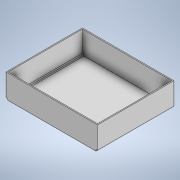
# Autodesk Inventor part: soap-collector
Saved by Autodesk Inventor 2020.2 (Build 242310000, 310)
## iProperties
Created: 2020-03-31
Part Number: soap-collector
Material: Generic
Document SubType Name: Modeling
Designer: iamin
Density: 1 g/cm^3
Appearance: Default
Author: iamin
Autodesk Inventor part; units mm, degrees
ref_plane "YZ Plane" through (0, 0, 0) normal (1, 0, 0) x (0, 1, 0)
ref_plane "XZ Plane" through (0, 0, 0) normal (0, 1, 0) x (-1, 0, 0)
ref_plane "XY Plane" through (0, 0, 0) normal (0, 0, 1) x (1, 0, 0)
sketch "Sketch1" plane through (0, 0, 0) normal (0, 0, 1) x (1, 0, 0)
  line L0 (-43.15, -11.5) -> (44.65, -11.5)
  line L1 (44.65, -11.5) -> (44.65, 11.5)
  line L2 (44.65, 11.5) -> (-44.65, 11.5)
  line L3 (-44.65, 11.5) -> (-44.65, -11.5)
  line L4 (-44.65, -11.5) -> (44.65, 11.5) construction
  line L5 (44.65, -11.5) -> (-44.65, 11.5) construction
  line L6 (-44.65, -11.5) -> (-44.65, -10)
  line L7 (-44.65, -10) -> (-43.15, -10)
  line L8 (-43.15, -10) -> (-43.15, -11.5)
  line L9 (0, 0) -> (0, -4.954)
  line L10 (44.65, -11.5) -> (-44.65, -11.5)
  line L11 (44.65, 11.5) -> (44.65, -11.5)
  line L12 (44.65, -11.5) -> (-44.65, 11.5) construction
  line L13 (44.65, -11.5) -> (44.65, -10)
  line L14 (44.65, -10) -> (43.15, -10)
  line L15 (43.15, -10) -> (43.15, -11.5)
  dimension "d0" = 89.3
  dimension "d1" = 23
  dimension "d3" = 1.5
  constraints: 32 end point, 7 symmetric about line, 3 perpendicular, 3 point on line, 2 midpoint, 2 parallel, 1 horizontal, 1 vertical
  measures "d0" distance of L2.end L1.end
  measures "d1" distance of L1.end L0.end
  measures "d3" distance of L6.end L7.end
extrude "Extrusion1" add sketch "Sketch1" along normal mid plane 74.55 contours L8 L7 L3 L2 L1 L14 L15 L0
shell "Shell1" thickness 1 removed faces 1 at (14.8833, 11.5, -12.425)
body "Solid1"
